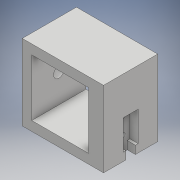
# Autodesk Inventor part: holder
Saved by Autodesk Inventor 2017 (Build 210142000, 142)
## iProperties
Created: 2018-04-15
Part Number: holder
Material: Generic
Document SubType Name: Modeling
Designer: dasae
Density: 1 g/cm^3
Appearance: Default
Author: dasae
Autodesk Inventor part; units mm, degrees
ref_plane "YZ Plane" through (0, 0, 0) normal (1, 0, 0) x (0, 1, 0)
ref_plane "XZ Plane" through (0, 0, 0) normal (0, 1, 0) x (-1, 0, 0)
ref_plane "XY Plane" through (0, 0, 0) normal (0, 0, 1) x (1, 0, 0)
sketch "Sketch1" plane through (0, 0, 0) normal (0, 1, 0) x (-1, 0, 0)
  line L0 (-10.5, -10.5) -> (10.5, -10.5)
  line L1 (10.5, -10.5) -> (10.5, 10.5)
  line L2 (10.5, 10.5) -> (-10.5, 10.5)
  line L3 (-10.5, 10.5) -> (-10.5, -10.5)
  line L4 (-10.5, -10.5) -> (10.5, 10.5) construction
  line L5 (10.5, -10.5) -> (-10.5, 10.5) construction
  line L6 (-14, -14) -> (14, -14)
  line L7 (14, -14) -> (14, 14)
  line L8 (14, 14) -> (-14, 14)
  line L9 (-14, -14) -> (14, 14) construction
  line L10 (14, -14) -> (-14, 14) construction
  line L11 (-14, 14) -> (-16, 14)
  line L12 (-14, -14) -> (-16, -14)
  line L13 (-16, -14) -> (-16, 14)
  line L14 (-14, 14) -> (-14, 10.5)
  line L15 (-14, -10.5) -> (-14, -14)
  point P0 (0, 0)
  dimension "d0" = 21
  dimension "d1" = 21
  dimension "d2" = 28
  dimension "d3" = 28
  dimension "d6" = 2
  constraints: 32 end point, 5 parallel, 4 horizontal, 4 midpoint, 3 perpendicular, 2 point on line
  measures "d0" distance of L2.end L1.end
  measures "d1" distance of L1.end L0.end
  measures "d2" distance of L8.end L7.end
  measures "d3" distance of L7.end L6.end
  measures "d6" distance of L8.end L11.end
extrude "Extrusion1" add sketch "Sketch1" along normal blind 20
sketch "Sketch3" plane through (16, 0, 14) normal (1, 0, 0) x (0, 0, -1)
  line L0 (28, 0) -> (28, 20) projected
  line L1 (28, 10) -> (0, 10) construction
  line L2 (0, 0) -> (0, 20) projected
  line L3 (14, 10) -> (14, 12.75)
  line L4 (14, 12.75) -> (25, 12.75)
  line L5 (14, 10) -> (14, 7.25)
  line L6 (14, 7.25) -> (25, 7.25)
  line L7 (28, 12.75) -> (28, 11.75)
  line L8 (28, 11.75) -> (25, 11.75)
  line L9 (25, 11.75) -> (25, 12.75)
  line L10 (25, 7.25) -> (25, 8.25)
  line L11 (25, 8.25) -> (28, 8.25)
  point P0 (14, 0)
  dimension "d7" = 2.75
  dimension "d8" = 2.75
  dimension "d9" = 1
  dimension "d10" = 3
  dimension "d11" = 1
  dimension "d23" = 1
  constraints: 20 end point, 6 point on line, 5 perpendicular, 3 midpoint, 1 vertical
  measures "d7" distance of L3.start L3.end
  measures "d8" distance of L3.start L5.end
  measures "d9" distance of L7.start L7.end
  measures "d10" distance of L7.end L8.end
  measures "d11" distance of L6.end L10.end
  measures "d23" distance of L8.end L4.end
extrude "Extrusion2" cut sketch "Sketch3" against normal blind 3
sketch "Sketch4" plane through (13, 0, 14) normal (1, 0, 0) x (0, 0, -1)
  line L0 (28, 11.75) -> (28, 8.25) projected
  line L1 (28, 10) -> (14, 10) construction
  circle A0 centre (22.5, 10) radius 0.95
  circle A1 centre (16.5, 10) radius 0.95
  line L2 (14, 7.25) -> (14, 12.75) projected
  point P0 (14, 0)
  dimension "d14" = 1.9
  dimension "d15" = 1.9
  dimension "d16" = 6
  dimension "d22" = 2.5
  constraints: 2 centre point, 2 end point, 2 point on line, 1 horizontal, 1 midpoint
  measures "d14" diameter of A0
  measures "d15" diameter of A1
  measures "d16" distance of A0.centre A1.centre
  measures "d22" distance from line of L2 A1.centre
extrude "Extrusion3" cut sketch "Sketch4" against normal blind 3
sketch "Sketch5" plane through (-14, 0, -14) normal (-1, 0, 0) x (0, 0, 1)
  line L0 (14, 7.25) -> (14, 12.75) projected
  circle A0 centre (14, 10) radius 1.95
  point P0 (14, 0)
  dimension "d19" = 3.9
  constraints: 1 centre point, 1 midpoint
  measures "d19" diameter of A0
extrude "Extrusion4" cut sketch "Sketch5" against normal blind 4
body "Solid1"
